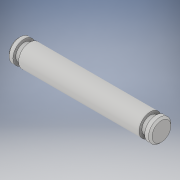
# Autodesk Inventor part: handle pivot pin
Saved by Autodesk Inventor 2017.1 (Build 211199000, 199)
## iProperties
Created: 2017-04-20
Part Number: handle pivot pin
Material: Generic
Document SubType Name: Modeling
Designer: 196918
Density: 1 g/cm^3
Appearance: Default
Author: 196918
Autodesk Inventor part; units mm, degrees
ref_plane "YZ Plane" through (0, 0, 0) normal (1, 0, 0) x (0, 1, 0)
sketch "Sketch1" plane through (0, 0, 0) normal (1, 0, 0) x (0, 1, 0)
  circle A0 centre (0, 0) radius 3.175
  dimension "d0" = 6.35
  constraints: 1 centre point, 1 coincident
  measures "d0" diameter of A0
extrude "Extrusion1" add sketch "Sketch1" along normal blind 40.4876
chamfer "Chamfer1" distance 0.508 angle 45 2 edges at (40.4876, -3.175, 0) (0, -3.175, 0)
ref_plane "Work Plane1" through (37.3126, 0, 0) normal (1, 0, 0) x (0, 0, -1)
sketch "Sketch2" plane through (37.3126, 0, 0) normal (1, 0, 0) x (0, 0, -1)
  circle A0 centre (0, 0) radius 2.3813
  circle A1 centre (0, 0) radius 3.175
  dimension "d7" = 4.7625
  constraints: 2 centre point, 2 coincident
  measures "d7" diameter of A0
extrude "Extrusion2" cut sketch "Sketch2" along normal blind 1.5875
ref_plane "Work Plane2" through (3.175, 0, 0) normal (-1, 0, 0) x (0, 0, 1)
sketch "Sketch3" plane through (3.175, 0, 0) normal (-1, 0, 0) x (0, 0, 1)
  circle A0 centre (0, 0) radius 2.3813
  circle A1 centre (0, 0) radius 3.175
  dimension "d11" = 4.7625
  constraints: 2 centre point, 2 coincident
  measures "d11" diameter of A0
extrude "Extrusion3" cut sketch "Sketch3" along normal blind 1.5875
body "Solid1"
